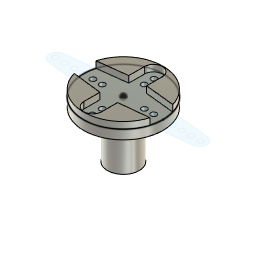
Servo_Horn2SALI v1 (Autodesk Fusion 360 design; units mm, degrees)
Autodesk Fusion 360 part; units mm, degrees
note: some values were not read from the file. Chosen so that the rebuilt part matches the saved one: which face or edge a step refers to. Set by a fixed rule: which sketch regions a step uses.
imported_body "基準フィーチャ1" makes body 1
sketch "スケッチ1" plane through (0, 0, 0) normal (0, 0, -1) x (1, 0, 0)
  circle A0 centre (16, 31.4974) radius 0.6
  circle A1 centre (8, 31.4974) radius 0.6
  circle A2 centre (14, 31.4974) radius 0.6
  circle A3 centre (18, 31.4974) radius 0.6
  circle A4 centre (10, 31.4974) radius 0.6
  circle A5 centre (12, 31.4974) radius 0.6
  circle A6 centre (20, 31.4908) radius 0.6
  line L0 (5.3664, 28.4028) -> (20, 29.9115)
  arc A7 (20, 29.9115) -> (20, 33.072) centre (19.75, 31.4917) ccw
  line L1 (20, 33.072) -> (5.3664, 34.5961)
  line L2 (5.3664, 34.5961) -> (5.3664, 38.0124)
  spline S0 degree 3 poles (5.3664, 38.0124) (5.3527, 38.1358) (5.3491, 38.386) (5.2324, 38.7443) (5.0571, 39.0746) (4.7402, 39.4615) (4.2135, 39.8145) (3.4672, 39.9614) (2.7211, 39.8144) (2.1944, 39.4614) (1.8776, 39.0744) (1.7021, 38.7442) (1.5862, 38.3857) (1.5806, 38.1357) (1.5664, 38.0124) knots -0.595957 -0.595957 -0.595957 -0.595957 -0.558709 -0.521462 -0.484215 -0.446967 -0.372473 -0.297978 -0.223484 -0.148989 -0.111742 -0.074495 -0.037247 0 0 0 0
  line L3 (1.5664, 38.0124) -> (1.5664, 34.5873)
  line L4 (1.5664, 34.5873) -> (-10.9393, 33.0969)
  arc A8 (-10.9393, 33.0969) -> (-10.9411, 29.9198) centre (-10.75, 31.5083) ccw
  line L5 (-10.9411, 29.9198) -> (1.5664, 28.4146)
  line L6 (1.5664, 28.4146) -> (1.5664, 25.0144)
  spline S1 degree 3 poles (1.5664, 25.0144) (1.5806, 24.8911) (1.5862, 24.6411) (1.7021, 24.2826) (1.8776, 23.9524) (2.1944, 23.5654) (2.7211, 23.2124) (3.4672, 23.0654) (4.2135, 23.2123) (4.7402, 23.5653) (5.0571, 23.9522) (5.2324, 24.2825) (5.3491, 24.6408) (5.3527, 24.891) (5.3664, 25.0144) knots -0.595956 -0.595956 -0.595956 -0.595956 -0.558709 -0.521462 -0.484215 -0.446967 -0.372473 -0.297978 -0.223484 -0.148989 -0.111742 -0.074495 -0.037247 0 0 0 0
  line L7 (5.3664, 25.0144) -> (5.3664, 28.4028)
  circle A9 centre (-1, 31.5026) radius 0.6
  circle A10 centre (-5, 31.5026) radius 0.6
  circle A11 centre (-7, 31.5026) radius 0.6
  circle A12 centre (-3, 31.5026) radius 0.6
  circle A13 centre (-11, 31.5026) radius 0.6
  circle A14 centre (-9, 31.5026) radius 0.6
  circle A15 centre (3.467, 24.8933) radius 0.6
  circle A16 centre (3.4673, 26.9933) radius 0.6
  circle A17 centre (3.4672, 36.0034) radius 0.6
  circle A18 centre (3.4674, 38.1035) radius 0.6
  arc A19 (5.3226, 29.6109) -> (5.2469, 33.4593) centre (3.5, 31.5) ccw
  line L8 (5.3226, 29.6109) -> (5.3226, 29.6109)
  arc A20 (5.2469, 33.4593) -> (5.3226, 29.6109) centre (3.5, 31.5) ccw
  circle A21 centre (3.5, 31.5) radius 8.5
  dimension "d131" = 17
  constraint concentric A20 A21
  measures "d131" diameter of A21
extrude "押し出し1" add sketch "スケッチ1" along normal blind 2 separate body contours A5 A21 | A5 L0 L1 L2 S0 L3 L4 L5 L6 S1 L7 A10 A21 | L1 L2 S0 L3 L4 A21 | L0 L5 L6 S1 L7 A21 | A10 A21 | A19 A20 picked at (11.8124, 31.3607) picked at (-4.7984, 31.5026) makes body 2
extrude "押し出し2" add sketch "スケッチ1" against normal blind 1.4 contours L1 L2 S0 L3 L4 A21 | L0 L5 L6 S1 L7 A21 bodies 2
sketch "スケッチ2" plane through (0, 0, -2) normal (0, 0, -1) x (1, 0, 0)
  circle A0 centre (10, 31.4974) radius 0.6
  circle A1 centre (-3, 31.5026) radius 0.6
  circle A2 centre (3.4673, 26.9933) radius 0.6
  circle A3 centre (3.467, 24.8933) radius 0.6
  circle A4 centre (3.4672, 36.0034) radius 0.6
  circle A5 centre (3.4674, 38.1035) radius 0.6
  circle A6 centre (-1, 31.5026) radius 0.6
  circle A7 centre (8, 31.4974) radius 0.6
  circle A8 centre (3.5, 31.5) radius 8.5
  circle A9 centre (3.5, 31.5) radius 1.4
  circle A10 centre (3.5, 31.5) radius 3.4
  dimension "d132" = 2.8
  dimension "d133" = 2
  constraint concentric A8 A9
  measures "d132" diameter of A9
extrude "押し出し3" add sketch "スケッチ2" along normal blind 10 contours A10 bodies 2
hidden bodies 1
named bodies: "Servo_Horn5"
